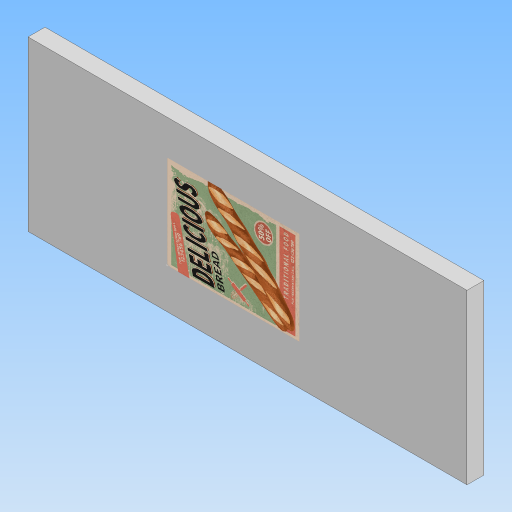
# Autodesk Inventor part: Part1
Saved by Autodesk Inventor 2024.2 (Build 282272000, 272)
## iProperties
Created: 2023-11-18
Part Number: Part1
Material: Generic
Document SubType Name: Modeling
Designer: MenMe
Density: 1 g/cm^3
Appearance: Default
Author: MenMe
Autodesk Inventor part; units mm, degrees
ref_plane "YZ Plane" through (0, 0, 0) normal (1, 0, 0) x (0, 1, 0)
ref_plane "XZ Plane" through (0, 0, 0) normal (0, 1, 0) x (-1, 0, 0)
ref_plane "XY Plane" through (0, 0, 0) normal (0, 0, 1) x (1, 0, 0)
sketch "Sketch1" plane through (0, 0, 0) normal (0, 0, 1) x (1, 0, 0)
  line L0 (0, 0) -> (259.5974, 0)
  line L1 (259.5974, 0) -> (259.5974, 99.6395)
  line L2 (259.5974, 99.6395) -> (0, 99.6395)
  line L3 (0, 99.6395) -> (0, 0)
  line L4 (97.5421, 88.1734) -> (173.2221, 88.1734) construction
  line L5 (173.2221, 88.1734) -> (173.2221, 12.4934) construction
  line L6 (173.2221, 12.4934) -> (97.5421, 12.4934) construction
  line L7 (97.5421, 12.4934) -> (97.5421, 88.1734) construction
  constraints: 8 end point, 2 parallel, 1 horizontal, 1 perpendicular, 2 other
extrude "Extrusion1" add sketch "Sketch1" along normal blind 10
sketch "Sketch2" plane through (0, 0, 10) normal (0, 0, 1) x (1, 0, 0)
  line L0 (77.4876, 7.3202) -> (77.4876, 94.5147) construction
  line L1 (77.4876, 94.5147) -> (164.6821, 94.5147) construction
  line L2 (164.6821, 94.5147) -> (164.6821, 7.3202) construction
  line L3 (164.6821, 7.3202) -> (77.4876, 7.3202) construction
  point P0 (0, 0)
  constraints: 2 other
decal "Decal1"
body "Solid1"
